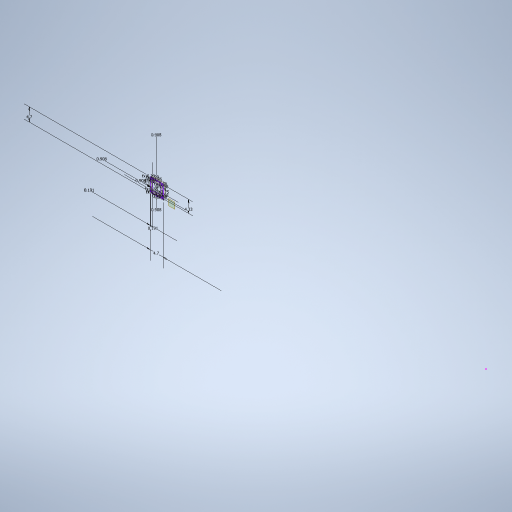
# Autodesk Inventor part: bracket
Saved by Autodesk Inventor 2024 (Build 280153000, 153)
## iProperties
Created: 2024-04-22
Part Number: bracket
Material: Generic
Document SubType Name: Modeling
Designer: Ruki
Density: 1 g/cm^3
Appearance: Default
Author: Ruki
Autodesk Inventor part; units mm, degrees
ref_plane "YZ Plane" through (0, 0, 0) normal (1, 0, 0) x (0, 1, 0)
ref_plane "XZ Plane" through (0, 0, 0) normal (0, 1, 0) x (-1, 0, 0)
ref_plane "XY Plane" through (0, 0, 0) normal (0, 0, 1) x (1, 0, 0)
ref_plane "Work Plane3" through (-1117.6, -50.8, 0) normal (0, 0, -1) x (-1, 0, 0)
sketch "Sketch1" plane through (-1117.6, -50.8, 0) normal (0, 0, -1) x (-1, 0, 0)
  line L0 (76.5714, 45.9614) -> (29.5714, 45.9614)
  line L1 (29.5714, 45.9614) -> (29.5714, -1.0386)
  line L2 (29.5714, -1.0386) -> (76.5714, -1.0386)
  line L3 (76.5714, -1.0386) -> (76.5714, 45.9614)
  circle A0 centre (71.7603, 41.2725) radius 1
  line L4 (74.6603, 44.1725) -> (31.3603, 44.1725)
  line L5 (31.3603, 44.1725) -> (31.3603, 0.8725)
  line L6 (31.3603, 0.8725) -> (74.6603, 0.8725)
  line L7 (74.6603, 0.8725) -> (74.6603, 44.1725)
  circle A1 centre (34.2603, 41.2725) radius 1
  circle A2 centre (34.2603, 3.7725) radius 1
  circle A3 centre (71.7603, 3.7725) radius 1
  line L8 (38.6492, 8.0392) -> (67.4936, 8.0392)
  line L9 (67.4936, 8.0392) -> (67.4936, 36.8837)
  line L10 (67.4936, 36.8837) -> (38.6492, 36.8837)
  line L11 (38.6492, 36.8837) -> (38.6492, 8.0392)
  line L12 (74.6603, 0.8725) -> (68.8603, 0.8725)
  line L13 (68.8603, 0.8725) -> (68.8603, 6.6725)
  line L14 (68.8603, 6.6725) -> (74.6603, 6.6725)
  line L15 (74.6603, 6.6725) -> (74.6603, 0.8725)
  line L16 (31.3603, 0.8725) -> (37.1603, 0.8725)
  line L17 (37.1603, 0.8725) -> (37.1603, 6.6725)
  line L18 (37.1603, 6.6725) -> (31.3603, 6.6725)
  line L19 (31.3603, 6.6725) -> (31.3603, 0.8725)
  line L20 (31.3603, 44.1725) -> (37.1603, 44.1725)
  line L21 (37.1603, 44.1725) -> (37.1603, 38.3725)
  line L22 (37.1603, 38.3725) -> (31.3603, 38.3725)
  line L23 (31.3603, 38.3725) -> (31.3603, 44.1725)
  line L24 (74.6603, 44.1725) -> (68.8603, 44.1725)
  line L25 (68.8603, 44.1725) -> (68.8603, 38.3725)
  line L26 (68.8603, 38.3725) -> (74.6603, 38.3725)
  line L27 (74.6603, 38.3725) -> (74.6603, 44.1725)
  point P0 (-1117.6, 50.8)
  point P1 (53.0714, 45.9614)
  point P2 (53.0714, -1.0386)
  point P3 (31.3603, 3.7725)
  point P4 (34.2603, 44.1725)
  point P5 (31.3603, 6.6725)
  point P6 (37.1603, 0.8725)
  point P7 (74.6603, 6.6725)
  point P8 (68.8603, 0.8725)
  point P9 (74.6603, 38.3725)
  point P10 (68.8603, 44.1725)
  point P11 (31.3603, 38.3725)
  point P12 (37.1603, 44.1725)
  dimension "d1" = 47
  dimension "d2" = 47
  dimension "d4" = 2
  dimension "d6" = 1.9111
  dimension "d7" = 1.9111
  dimension "d8" = 43.3
  dimension "d9" = 43.3
  dimension "d10" = 2
  dimension "d14" = 2
  dimension "d17" = 2
  dimension "d24" = 9.0778
  dimension "d25" = 9.0778
  dimension "d26" = 9.0778
  dimension "d27" = 9.0778
  dimension "d61" = 5.8
  dimension "d62" = 5.8
  dimension "d63" = 5.8
  dimension "d64" = 5.8
  dimension "d65" = 5.8
  dimension "d66" = 5.8
  dimension "d67" = 5.8
  dimension "d68" = 5.8
  dimension "d69" = 37.5
  dimension "d70" = 37.5
  dimension "d71" = 37.5
  dimension "d72" = 37.5
  dimension "d73" = 2.9
  dimension "d74" = 2.9
  constraints: 56 end point, 14 parallel, 7 horizontal, 7 perpendicular, 4 centre point, 4 midpoint
  measures "d1" distance of point (53.071, 45.961) point (53.071, -1.039)
  measures "d2" distance between parallel lines of L1 L3
  measures "d4" diameter of A0
  measures "d6" distance between parallel lines of L3 L7
  measures "d7" distance between parallel lines of L2 L6
  measures "d8" distance between parallel lines of L5 L7
  measures "d9" distance between parallel lines of L6 L4
  measures "d10" diameter of A1
  measures "d14" diameter of A2
  measures "d17" diameter of A3
  measures "d24" distance between parallel lines of L1 L11
  measures "d25" distance between parallel lines of L3 L9
  measures "d26" distance between parallel lines of L2 L8
  measures "d27" distance between parallel lines of L0 L10
  measures "d61" distance of L24.end L25.end
  measures "d62" distance between parallel lines of L7 L25
  measures "d63" distance between parallel lines of L7 L13
  measures "d64" distance between parallel lines of L6 L14
  measures "d65" distance from line of point (31.36, 3.773) L17
  measures "d66" distance between parallel lines of L6 L18
  measures "d67" distance from line of point (34.26, 44.173) L22
  measures "d68" distance between parallel lines of L5 L21
  measures "d69" distance of A0.centre A3.centre
  measures "d70" distance of A2.centre A3.centre
  measures "d71" distance of A1.centre A2.centre
  measures "d72" distance of A1.centre A0.centre
  measures "d73" distance from line of L7 A0.centre
  measures "d74" distance from line of L4 A0.centre
extrude "Extrusion3" add sketch "Sketch1" along normal blind 8 contours L3 L2 L1 L0
extrude "Extrusion7" add sketch "Sketch1" along normal blind 3 contours L7 L26 L25 L4 | L21 L22 L5 L4 | L7 L6 L13 L14 | L18 L17 L6 L5
extrude "Extrusion8" add sketch "Sketch1" against normal blind 1 contours L3 L2 L1 L0 | A0 | L7 L26 L25 L4 | L25 L26 L7 L14 L13 L6 L17 L18 L5 L22 L21 L4 | L21 L22 L5 L4 | L7 L6 L13 L14 | L18 L17 L6 L5 | A1 | A2 | A3
extrude "Extrusion6" cut sketch "Sketch1" along normal mid plane 10 contours A0 | A1 | A2 | A3
fillet "Fillet5" radius 10 4 edges at (-1156.2492, -13.9163, 0.5) (-1185.0936, -13.9163, 0.5) (-1185.0936, -42.7608, 0.5) (-1156.2492, -42.7608, 0.5)
fillet "Fillet6" radius 2 4 edges at (-1194.1714, -4.8386, -3.5) (-1147.1714, -4.8386, -3.5) (-1194.1714, -51.8386, -3.5) (-1147.1714, -51.8386, -3.5)
fillet "Fillet7" radius 4 4 edges at (-1154.7603, -12.4275, -1.5) (-1186.4603, -12.4275, -1.5) (-1186.4603, -44.1275, -1.5) (-1154.7603, -44.1275, -1.5)
equation "\"d10\" = d4"
equation "\"d14\" = d4"
equation "\"d17\" = d4"
equation "\"d61\" = 2 * d73"
equation "\"d73\" = -0.5 * d72 + 0.5 * d8"
body "Solid2"
